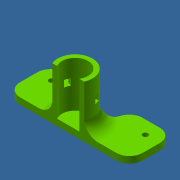
# Autodesk Inventor part: WristCableHolder
Saved by Autodesk Inventor 2016 (Build 200138000, 138)
## iProperties
Created: 2015-09-24
Part Number: WristCableHolder
Material: ABS-Kunststoff
Document SubType Name: Modeling
Designer: 4ndreas
Density: 1.06 g/cm^3
Appearance: Glatt - grün
Mass: 4.45496 g
Surface Area: 36.5385 cm^2
Volume: 4.20279 cm^3
Author: 4ndreas
Autodesk Inventor part; units mm, degrees
ref_plane "YZ Plane" through (0, 0, 0) normal (1, 0, 0) x (0, 1, 0)
ref_plane "XZ Plane" through (0, 0, 0) normal (0, 1, 0) x (-1, 0, 0)
ref_plane "XY Plane" through (0, 0, 0) normal (0, 0, 1) x (1, 0, 0)
sketch "Skizze1" plane through (0, 0, 0) normal (0, 0, 1) x (1, 0, 0)
  circle A0 centre (8.096, 35.908) radius 1.25 projected
  circle A1 centre (51.26, 35.908) radius 1.25 projected
  arc A2 (12.3473, 60.8404) -> (11.3298, 70.3413) centre (5.4583, 64.9075) ccw projected
  arc A3 (53.1253, 78.6488) -> (11.3298, 70.3413) centre (29.678, 87.322) ccw projected
  line L0 (53.1253, 78.6488) -> (38.588, 39.3481) projected
  arc A4 (20.1802, 42.8448) -> (38.588, 39.3481) centre (29.678, 42.6439) ccw projected
  arc A5 (20.1802, 42.8448) -> (15.6007, 50.2467) centre (12.1819, 43.014) ccw projected
  arc A6 (12.3473, 60.8404) -> (15.6007, 50.2467) centre (18.8057, 57.0274) ccw projected
  line L1 (8.096, 25) -> (51.26, 25) projected
  line L2 (51.26, 25) -> (51.26, 0) projected
  line L3 (59.3561, 0) -> (51.26, 0) projected
  line L4 (59.3561, 0) -> (59.3561, 87.322) projected
  arc A7 (59.3561, 87.322) -> (0, 87.322) centre (29.678, 87.322) ccw projected
  line L5 (0, 0) -> (0, 87.322) projected
  line L6 (8.096, 0) -> (0, 0) projected
  line L7 (8.096, 0) -> (8.096, 25) projected
  line L8 (57.8561, 22) -> (57.8561, 42)
  line L9 (57.8561, 42) -> (39.5689, 42)
  line L10 (39.5689, 42) -> (36.2931, 33.1439)
  line L11 (36.2931, 33.1439) -> (23.063, 33.1439)
  line L12 (23.063, 33.1439) -> (19.7871, 42)
  line L13 (19.7871, 42) -> (1.5, 42)
  line L14 (1.5, 42) -> (1.5, 22)
  line L15 (1.5, 22) -> (57.8561, 22)
  line L16 (29.678, 87.322) -> (29.678, 42.6439) construction
  dimension "d0" = 1.5
  dimension "d1" = 3
  dimension "d2" = 20
  constraints: 18 end point, 2 perpendicular, 2 tangent, 2 vertical, 1 collinear, 1 parallel, 1 symmetric about line, 3 other
  measures "d0" distance between parallel lines of L8 L4
  measures "d1" distance between parallel lines of L1 L15
  measures "d2" distance between parallel lines of L15 L9
extrude "Extrusion1" add sketch "Skizze1" along normal blind 3 contours L9 L8 L15 L2 L1 L7 L14 L13 L12 L11 L10 L0 | L15 L7 L1 L2
sketch "Skizze2" plane through (0, 0, 3) normal (0, 0, 1) x (1, 0, 0)
  circle A0 centre (51.26, 35.908) radius 1.25 construction
  circle A1 centre (8.096, 35.908) radius 1.25 construction
  line L0 (57.8561, 22) -> (57.8561, 42) construction
  line L1 (57.8561, 42) -> (39.5689, 42) construction
  line L2 (39.5689, 42) -> (36.2931, 33.1439) construction
  line L3 (36.2931, 33.1439) -> (23.063, 33.1439) construction
  line L4 (23.063, 33.1439) -> (19.7871, 42) construction
  line L5 (19.7871, 42) -> (1.5, 42) construction
  line L6 (1.5, 42) -> (1.5, 22) construction
  line L7 (1.5, 22) -> (57.8561, 22)
  arc A2 (37.0344, 22) -> (22.3217, 22) centre (29.678, 25.1439) ccw
  line L8 (36.2931, 33.1439) -> (23.063, 33.1439) projected
  line L9 (29.678, 22) -> (29.678, 33.1439) construction
  line L10 (1.5, 22) -> (57.8561, 22)
  arc A3 (34.7884, 22) -> (24.5677, 22) centre (29.678, 25.1439) ccw
  line L11 (34.7884, 22) -> (37.0344, 22)
  line L12 (24.5677, 22) -> (22.3217, 22)
  point P0 (0, 0)
  dimension "d5" = 2
  dimension "d6" = 8
  constraints: 10 end point, 5 point on line, 4 point on circle, 3 midpoint, 2 centre point, 2 collinear, 1 coincident, 1 tangent
  measures "d5" radial gap between concentric circles of A3 A2
  measures "d6" radius of A2
extrude "Extrusion2" add sketch "Skizze2" along normal blind 10 contours A2 L7 A3
fillet "Rundung1" radius 6 10 edges at (23.0015, 29.5512, 3) (36.3545, 29.5512, 3) (1.5, 42, 1.5) (1.5, 22, 1.5) (19.7871, 42, 1.5) (23.063, 33.1439, 1.5) (36.2931, 33.1439, 1.5) (39.5689, 42, 1.5) (57.8561, 42, 1.5) (57.8561, 22, 1.5)
sketch "Skizze3" plane through (0, 0, 13) normal (0, 0, 1) x (1, 0, 0)
  arc A0 (34.7884, 22) -> (24.5677, 22) centre (29.678, 25.1439) ccw projected
  line L0 (34.7884, 22) -> (37.0344, 22) projected
  arc A1 (37.0344, 22) -> (22.3217, 22) centre (29.678, 25.1439) ccw projected
  line L1 (22.3217, 22) -> (24.5677, 22) projected
  line L2 (37.5308, 26.6719) -> (35.62, 25.9764)
  line L3 (34.7649, 28.3256) -> (36.6757, 29.0211)
  line L4 (29.678, 25.1439) -> (29.678, 31.1439) construction
  line L5 (29.678, 25.1439) -> (37.1956, 27.8801) construction
  line L6 (24.5911, 28.3256) -> (22.6803, 29.0211)
  line L7 (23.7361, 25.9764) -> (21.8253, 26.6719)
  point P0 (0, 0)
  dimension "d10" = 2.5
  dimension "d11" = 70
  constraints: 12 end point, 10 point on circle, 1 parallel, 1 vertical, 3 other
  measures "d10" distance between parallel lines of L3 L2
  measures "d11" angle of L4 L5
extrude "Extrusion3" add sketch "Skizze3" along normal blind 3 contours A0 L2 A1 L0 | A0 L6 A1 L3 | A0 L1 A1 L7
sketch "Skizze4" plane through (0, 0, 16) normal (0, 0, 1) x (1, 0, 0)
  line L0 (21.8253, 26.6719) -> (23.7361, 25.9764) projected
  arc A0 (24.5911, 28.3256) -> (23.7361, 25.9764) centre (29.678, 25.1439) ccw projected
  line L1 (24.5911, 28.3256) -> (22.6803, 29.0211) projected
  arc A1 (22.6803, 29.0211) -> (21.8253, 26.6719) centre (29.678, 25.1439) ccw projected
  arc A2 (23.7361, 25.9764) -> (24.5677, 22) centre (29.678, 25.1439) ccw projected
  line L2 (23.7361, 25.9764) -> (21.8253, 26.6719) projected
  arc A3 (21.8253, 26.6719) -> (22.3217, 22) centre (29.678, 25.1439) ccw projected
  line L3 (22.3217, 22) -> (24.5677, 22) projected
  line L4 (34.7649, 28.3256) -> (36.6757, 29.0211) projected
  arc A4 (36.6757, 29.0211) -> (22.6803, 29.0211) centre (29.678, 25.1439) ccw projected
  line L5 (22.6803, 29.0211) -> (24.5911, 28.3256) projected
  arc A5 (34.7649, 28.3256) -> (24.5911, 28.3256) centre (29.678, 25.1439) ccw projected
  line L6 (35.62, 25.9764) -> (37.5308, 26.6719) projected
  arc A6 (37.5308, 26.6719) -> (36.6757, 29.0211) centre (29.678, 25.1439) ccw projected
  line L7 (36.6757, 29.0211) -> (34.7649, 28.3256) projected
  arc A7 (35.62, 25.9764) -> (34.7649, 28.3256) centre (29.678, 25.1439) ccw projected
  line L8 (34.7884, 22) -> (37.0344, 22) projected
  arc A8 (37.0344, 22) -> (37.5308, 26.6719) centre (29.678, 25.1439) ccw projected
  line L9 (37.5308, 26.6719) -> (35.62, 25.9764) projected
  arc A9 (34.7884, 22) -> (35.62, 25.9764) centre (29.678, 25.1439) ccw projected
  point P0 (0, 0)
extrude "Extrusion4" add sketch "Skizze4" along normal blind 8
